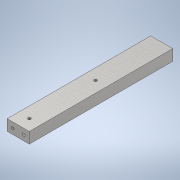
# Autodesk Inventor part: chair support
Saved by Autodesk Inventor 2022 (Build 260153000, 153)
## iProperties
Created: 2021-12-06
Part Number: chair support
Material: Generic
Document SubType Name: Modeling
Designer: Vedic
Density: 1 g/cm^3
Appearance: Default
Author: Vedic
Autodesk Inventor part; units mm, degrees
ref_plane "YZ Plane" through (0, 0, 0) normal (1, 0, 0) x (0, 1, 0)
ref_plane "XZ Plane" through (0, 0, 0) normal (0, 1, 0) x (-1, 0, 0)
ref_plane "XY Plane" through (0, 0, 0) normal (0, 0, 1) x (1, 0, 0)
sketch "Sketch1" plane through (0, 0, 0) normal (0, 1, 0) x (-1, 0, 0)
  line L0 (28.8109, 92.1657) -> (-21.9891, 92.1657)
  line L1 (-21.9891, 92.1657) -> (-21.9891, -238.0343)
  line L2 (-21.9891, -238.0343) -> (28.8109, -238.0343)
  line L3 (28.8109, -238.0343) -> (28.8109, 92.1657)
  point P0 (0, 0)
  dimension "d0" = 50.8
  dimension "d1" = 330.2
  constraints: 8 end point, 2 parallel, 1 horizontal, 1 perpendicular
  measures "d0" distance of L0.start L0.end
  measures "d1" distance of L2.end L0.start
extrude "Extrusion1" add sketch "Sketch1" along normal blind 25.4
sketch "Sketch2" plane through (-28.8109, 0, 92.1657) normal (0, 0, 1) x (1, 0, 0)
  line L0 (0, 0) -> (0, 25.4) projected
  line L1 (0, 12.7) -> (50.8, 12.7) construction
  line L2 (50.8, 0) -> (50.8, 25.4) projected
  circle A0 centre (12.7, 12.7) radius 3.175
  circle A1 centre (38.1, 12.7) radius 3.175
  line L3 (50.8, 25.4) -> (0, 25.4) construction
  line L4 (25.4, 25.4) -> (25.4, 0) construction
  line L5 (50.8, 0) -> (0, 0) construction
  point P0 (28.8109, 0)
  dimension "d4" = 6.35
  dimension "d5" = 6.35
  dimension "d6" = 12.7
  dimension "d7" = 12.7
  constraints: 4 end point, 4 midpoint, 2 centre point, 2 point on line
  measures "d4" diameter of A0
  measures "d5" diameter of A1
  measures "d6" distance from line of L4 A0.centre
  measures "d7" distance from line of L4 A1.centre
extrude "Extrusion2" cut sketch "Sketch2" against normal blind 25.4
sketch "Sketch3" plane through (21.9891, 0, -238.0343) normal (0, 0, -1) x (-1, 0, 0)
  line L0 (0, 0) -> (0, 25.4) construction
  line L1 (0, 12.7) -> (50.8, 12.7) construction
  line L2 (50.8, 0) -> (50.8, 25.4) construction
  line L3 (50.8, 25.4) -> (0, 25.4) construction
  line L4 (25.4, 25.4) -> (25.4, 0) construction
  line L5 (50.8, 0) -> (0, 0) construction
  circle A0 centre (12.7, 12.7) radius 3.175 projected
  circle A1 centre (12.7, 12.7) radius 3.175 construction
  circle A2 centre (38.1, 12.7) radius 3.175 projected
  circle A3 centre (38.1, 12.7) radius 3.175 construction
  point P0 (21.9891, 0)
  constraints: 4 end point, 4 midpoint, 2 centre point, 2 coincident
extrude "Extrusion3" cut sketch "Sketch3" against normal blind 25.4
sketch "Sketch4" plane through (0, 25.4, 0) normal (0, 1, 0) x (1, 0, 0)
  line L0 (-28.8109, -92.1657) -> (21.9891, -92.1657) construction
  line L1 (-3.4109, -92.1657) -> (-3.4109, 238.0343) construction
  line L2 (21.9891, 238.0343) -> (-28.8109, 238.0343) construction
  line L3 (-28.8109, 238.0343) -> (-28.8109, -92.1657) construction
  line L4 (-28.8109, 72.9343) -> (21.9891, 72.9343) construction
  line L5 (21.9891, -92.1657) -> (21.9891, 238.0343) construction
  circle A0 centre (-3.4109, -66.7657) radius 3.175
  circle A1 centre (-3.4109, 85.6343) radius 3.175
  point P0 (0, 0)
  dimension "d12" = 6.35
  dimension "d13" = 152.4
  dimension "d14" = 25.4
  constraints: 4 end point, 4 midpoint, 2 centre point, 2 point on line, 1 equal radius
  measures "d12" diameter of A1
  measures "d13" distance of A1.centre A0.centre
  measures "d14" distance from line of L0 A0.centre
extrude "Extrusion4" cut sketch "Sketch4" against normal through all
body "Solid1"
